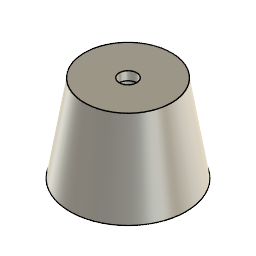
Wire Cutter Base Stand (Autodesk Fusion 360 design; units mm, degrees)
part number: 2025-10-24-17-21-36-739
Autodesk Fusion 360 part; units mm, degrees
sketch "Sketch1" plane through (0, 0, 0) normal (0, 0, 1) x (1, 0, 0)
  circle A0 centre (0, 0) radius 20
  dimension "d1" = 40
  constraint coincident A0.centre origin
  measures "d1" diameter of A0
ref_plane "WorkPlane1" through (0, 0, 30) normal (0, 0, 1) x (1, 0, 0)
sketch "Sketch2" plane through (0, 0, 30) normal (0, 0, 1) x (1, 0, 0)
  circle A0 centre (0, 0) radius 15
  dimension "d3" = 30
  constraint coincident A0.centre origin
  measures "d3" diameter of A0
loft "Loft1" add profiles "Sketch2", "Sketch1" section 1 section 2
sketch "Sketch3" plane through (0, 0, 0) normal (0, 0, -1) x (1, 0, 0)
  circle A0 centre (0, 0) radius 20
  circle A1 centre (0, 0) radius 7.5
  dimension "d4" = 15
  constraint coincident A0.centre A1.centre
  measures "d4" diameter of A1
extrude "Extrude1" cut sketch "Sketch3" against normal blind 27 contours A1
sketch "Sketch4" plane through (0, 0, 27) normal (0, 0, -1) x (1, 0, 0)
  circle A0 centre (0, 0) radius 7.5
  circle A1 centre (0, 0) radius 3
  dimension "d7" = 6
  constraint coincident A0.centre A1.centre
  measures "d7" diameter of A1
extrude "Extrude2" cut sketch "Sketch4" against normal blind 7 contours A1
